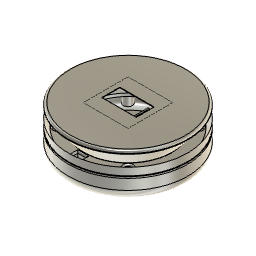
IR Hub v26 (Autodesk Fusion 360 design; units mm, degrees)
Autodesk Fusion 360 part; units mm, degrees
note: some values were not read from the file. Set by a fixed rule: which sketch regions a step uses.
sketch "Sketch1" plane through (0, 0, 0) normal (0, 1, 0) x (1, 0, 0)
  line L0 (0, 0) -> (0, -2) construction
  line L1 (0, -2) -> (33, -2)
  line L2 (38, -7) -> (38, -14)
  line L3 (0, -2) -> (0, 0)
  line L4 (38, -14) -> (40, -14)
  arc A0 (38, -7) -> (33, -2) centre (33, -7) ccw
  line L5 (0, 0) -> (33, 0)
  arc A1 (40, -7) -> (33, 0) centre (33, -7) ccw
  line L6 (40, -7) -> (40, -14)
  line L7 (0, 0) -> (80, 0)
  line L8 (80, 0) -> (80, -14)
  line L9 (40, -14) -> (80, -14)
  point P0 (38, -2)
  dimension "d5" = 2
  dimension "d6" = 38
  dimension "d7" = 12
  dimension "d9" = 5
  dimension "d40" = 80
  dimension "d41" = 14
  constraint coincident L0.start L3.end
  constraint vertical L0
  constraint perpendicular L0 L1
  constraint perpendicular L1 L2
  constraint perpendicular L3 L5
  constraint perpendicular L4 L6
  constraint coincident P0 L1
  constraint coincident P0 L2
  constraint tangent L1 A0
  constraint tangent L2 A0
  constraint perpendicular L3 L7
  constraint perpendicular L5 L8
  measures "d5" distance of L0.start L0.end
  measures "d6" distance of L0.end P0
  measures "d7" distance of P0 L2.end
  measures "d9" radius of A0
  measures "d40" distance of L0.start L7.end
  measures "d41" distance of L7.end L8.end
revolve "Revolve1" add sketch "Sketch1" angle 360 about axis through (0, 0, 1.75) along (0, 0, 1) contours L1 L2 L3 L4 A0 L5 A1 L6 L7 makes body 1
sketch "Sketch2" plane through (0, 0, 2) normal (0, 0, 1) x (-1, 0, 0)
  circle A0 centre (0, 0) radius 33
  line L0 (-16, -29.5) -> (16, -29.5)
  line L1 (16, -29.5) -> (16, 29.5)
  line L2 (16, 29.5) -> (-16, 29.5)
  line L3 (-16, 29.5) -> (-16, -29.5)
  line L4 (-16, -29.5) -> (16, 29.5) construction
  line L5 (16, -29.5) -> (-16, 29.5) construction
  line L6 (-17, 30.5) -> (-17, -30.5)
  line L7 (-17, -30.5) -> (17, -30.5)
  line L8 (17, -30.5) -> (17, 30.5)
  line L9 (17, 30.5) -> (-17, 30.5)
  dimension "d16" = 32
  dimension "d17" = 59
  dimension "d20" = 1
  constraint horizontal L0
  constraint perpendicular L0 L1
  constraint parallel L0 L2
  constraint parallel L1 L3
  constraint coincident L4 A0.centre
  constraint coincident L5 A0.centre
  constraint coincident A0.centre origin
  measures "d16" distance of L1.end L2.end
  measures "d17" distance of L0.end L1.end
extrude "Extrude1" add sketch "Sketch2" along normal blind 1 contours A0 L1 L8 | A0 L1 L2 L8 L9 | A0 L0 L1 L7 L8 | A0 L2 L9 | A0 L0 L7 | A0 L2 L3 L6 L9 | A0 L0 L3 L6 L7 | A0 L3 L6 bodies 1
sketch "Sketch3" plane through (0, 30.5, 0) normal (0, 1, 0) x (-1, 0, 0)
  line L0 (17, 3) -> (-17, 3)
  line L1 (0, 2) -> (0, 5.5) construction
  line L2 (4.5, 7.5) -> (-4.5, 7.5)
  line L3 (-4.5, 7.5) -> (-4.5, 3.5)
  line L4 (-4.5, 3.5) -> (4.5, 3.5)
  line L5 (4.5, 3.5) -> (4.5, 7.5)
  line L6 (4.5, 7.5) -> (-4.5, 3.5) construction
  line L7 (-4.5, 7.5) -> (4.5, 3.5) construction
  line L8 (7.5, 9.5) -> (-7.5, 9.5)
  line L9 (-7.5, 9.5) -> (-7.5, 1.5)
  line L10 (-7.5, 1.5) -> (7.5, 1.5)
  line L11 (7.5, 1.5) -> (7.5, 9.5)
  line L12 (7.5, 9.5) -> (-7.5, 1.5) construction
  line L13 (-7.5, 9.5) -> (7.5, 1.5) construction
  line L14 (8.5, 1.5) -> (8.5, 10.5)
  line L15 (8.5, 10.5) -> (-8.5, 10.5)
  line L16 (-8.5, 10.5) -> (-8.5, 1.5)
  line L17 (-8.5, 1.5) -> (-7.5, 1.5)
  line L18 (8.5, 1.5) -> (7.5, 1.5)
  spline S0 degree 3 poles (17, 2.3824) (16.4779, 2.2768) (15.935, 2.1958) (14.4367, 2.0345) (13.4748, 2) (12.5996, 2) knots -1.596795 -1.596795 -1.596795 -1.596795 -1.446279 -1.446279 -1.183716 -1.183716 -1.183716 -1.183716
  line L19 (17, 2.3824) -> (17, 3)
  line L20 (-17, 3) -> (-17, 2.3824)
  spline S1 degree 3 poles (-12.5996, 2) (-13.4748, 2) (-14.4367, 2.0345) (-15.935, 2.1958) (-16.4779, 2.2768) (-17, 2.3824) knots 1.183716 1.183716 1.183716 1.183716 1.446279 1.446279 1.596795 1.596795 1.596795 1.596795
  line L21 (-12.5996, 2) -> (12.5996, 2)
  point P0 (0, 5.5)
  point P1 (0, 5.5)
  dimension "d23" = 3.5
  dimension "d24" = 9
  dimension "d25" = 4
  dimension "d29" = 15
  dimension "d30" = 8
  dimension "d31" = 1
  constraint perpendicular L0 L1
  constraint horizontal L2
  constraint perpendicular L2 L3
  constraint parallel L2 L4
  constraint parallel L3 L5
  constraint coincident L6 P1
  constraint coincident L7 P1
  constraint coincident P1 P0
  constraint horizontal L8
  constraint perpendicular L8 L9
  constraint parallel L8 L10
  constraint parallel L9 L11
  constraint coincident L12 P1
  constraint coincident L13 P1
  constraint perpendicular L9 L17
  constraint perpendicular L11 L18
  measures "d23" distance of L1.start P1
  measures "d24" distance of L3.end L4.end
  measures "d25" distance of L2.end L3.end
  measures "d29" distance of L9.end L10.end
  measures "d30" distance of L8.end L9.end
extrude "Extrude2" cut sketch "Sketch3" along normal blind 80 contours L0 L9 L11 L21 | L0 L8 L9 L11 | L9 L10 L11 L21 | L2 L3 L4 L5 bodies 1
extrude "Extrude3" add sketch "Sketch3" along normal blind 16.314 contours L0 L11 L14 L21 | L0 L8 L9 L11 L14 L15 L16 | L0 L9 L16 L21 bodies 1
extrude "Extrude4" add sketch "Sketch3" along normal blind 1 separate body contours L0 L8 L9 L11 makes body 2
extrude "Extrude5" add 1 faces at (-2.5, 30.5, 2) along direction (0, 1, 0) blind 1 on bodies 1 bodies 1 2
revolve "Revolve2" cut sketch "Sketch1" angle 360 about axis through (0, 0, 1.75) along (0, 0, 1) contours A1 L6 L7 L8 L9 bodies 1
sketch "Sketch4" plane through (0, 0, 0) normal (0, 0, 1) x (1, 0, 0)
  circle A0 centre (0, 0) radius 40
  circle A1 centre (0, 0) radius 37.6
  circle A2 centre (0, 0) radius 36.6
  line L0 (23.5, 23.5) -> (-23.5, 23.5) construction
  line L1 (-23.5, 23.5) -> (-23.5, -23.5) construction
  line L2 (-23.5, -23.5) -> (23.5, -23.5) construction
  line L3 (23.5, -23.5) -> (23.5, 23.5) construction
  line L4 (23.5, 23.5) -> (-23.5, -23.5) construction
  line L5 (-23.5, 23.5) -> (23.5, -23.5) construction
  circle A3 centre (23.5, 23.5) radius 2.5
  circle A4 centre (23.5, -23.5) radius 2.5
  circle A5 centre (-23.5, -23.5) radius 2.5
  circle A6 centre (-23.5, 23.5) radius 2.5
  circle A7 centre (-23.5, 23.5) radius 3
  circle A8 centre (23.5, 23.5) radius 3
  circle A9 centre (23.5, -23.5) radius 3
  circle A10 centre (-23.5, -23.5) radius 3
  line L6 (0, 0) -> (0, -33.234) construction
  line L7 (2.75, -30.984) -> (-2.75, -30.984)
  line L8 (-2.75, -30.984) -> (-2.75, -35.484)
  line L9 (-2.75, -35.484) -> (2.75, -35.484)
  line L10 (2.75, -35.484) -> (2.75, -30.984)
  line L11 (2.75, -30.984) -> (-2.75, -35.484) construction
  line L12 (-2.75, -30.984) -> (2.75, -35.484) construction
  line L13 (-3.25, -30.484) -> (-3.25, -35.984)
  line L14 (-3.25, -35.984) -> (3.25, -35.984)
  line L15 (3.25, -35.984) -> (3.25, -30.484)
  line L16 (3.25, -30.484) -> (-3.25, -30.484)
  circle A11 centre (0, 0) radius 29.5
  point P0 (0, -33.234)
  dimension "d43" = 80
  dimension "d50" = 47
  dimension "d51" = 47
  dimension "d53" = 5
  dimension "d54" = 5
  dimension "d55" = 5
  dimension "d56" = 5
  dimension "d58" = 0.5
  dimension "d59" = 0.5
  dimension "d60" = 0.5
  dimension "d61" = 0.5
  dimension "d65" = 33.234
  dimension "d66" = 5.5
  dimension "d67" = 4.5
  dimension "d68" = 0.5
  dimension "d70" = 59
  constraint coincident A0.centre A1.centre
  constraint horizontal L0
  constraint perpendicular L0 L1
  constraint parallel L0 L2
  constraint parallel L1 L3
  constraint coincident L4 A0.centre
  constraint coincident L5 A0.centre
  constraint coincident L0.start L3.end
  constraint coincident L2.end L3.start
  constraint coincident L1.end L2.start
  constraint coincident L0.end L1.start
  constraint vertical L6
  constraint horizontal L7
  constraint perpendicular L7 L8
  constraint parallel L7 L9
  constraint parallel L8 L10
  constraint coincident L11 P0
  constraint coincident L12 P0
  constraint coincident P0 L6.end
  measures "d43" diameter of A0
  measures "d50" distance of L1.end L2.end
  measures "d51" distance of L0.end L1.end
  measures "d53" diameter of A3
  measures "d54" diameter of A4
  measures "d55" diameter of A5
  measures "d56" diameter of A6
  measures "d65" distance of A0.centre P0
  measures "d66" distance of L8.end L9.end
  measures "d67" distance of L7.end L8.end
  measures "d70" diameter of A11
extrude "Extrude6" add sketch "Sketch4" along normal blind 1.5 separate body contours A0 | A1 | A2 makes body 3
extrude "Extrude7" add sketch "Sketch4" along normal blind 2.5 contours A1 bodies 3
extrude "Extrude8" add sketch "Sketch4" along normal blind 9.5 contours A7 | A8 | A9 | A10 bodies 3
extrude "Extrude9" add sketch "Sketch4" along normal blind 9.5 contours L13 L14 L15 L16 bodies 3
fillet "Fillet1" radius 1 8 edges at (21.1692, 24.404, 0) (21.1692, -22.596, 0) (0, -30.984, 0) (-2.75, -33.234, 0) (0, -35.484, 0) (2.75, -33.234, 0) (-25.8308, -22.596, 0) (-25.8308, 24.404, 0) on bodies 3
fillet "Fillet2" radius 0.5 1 edges at (-37.2931, -14.4646, 0) on bodies 3
sketch "Sketch5" plane through (0, 0, 0) normal (0, 1, 0) x (1, 0, 0)
  line L0 (0, 0) -> (29.5, 0) construction
  line L1 (29.5, 0) -> (40, -12.5134)
  line L2 (29.5, 0) -> (37.5, 0) construction
  line L3 (29.5, 0) -> (29, 0)
  line L4 (29, 0) -> (29, 2)
  line L5 (40, -12.5134) -> (40, 0) construction
  line L6 (40, -12.5134) -> (38.5, -12.5134)
  line L7 (38.5, -12.5134) -> (28, 0)
  line L8 (38.5, -12.5134) -> (60.6777, -12.5134) construction
  line L9 (28, 0) -> (28, 2)
  line L10 (28, 2) -> (29, 2)
  dimension "d88" = 29.5
  dimension "d89" = 50
  dimension "d90" = 16.3351
  dimension "d93" = 0.5
  dimension "d95" = 2
  dimension "d97" = 1.5
  dimension "d98" = 130
  dimension "d99" = 2
  constraint coincident L0.start origin
  constraint horizontal L0
  constraint horizontal L2
  constraint parallel L0 L3
  constraint perpendicular L0 L4
  constraint horizontal L6
  constraint perpendicular L5 L6
  constraint horizontal L8
  constraint coincident L0 L7.end
  constraint perpendicular L0 L9
  measures "d88" distance of L0.start L0.end
  measures "d89" angle of L1 L2
  measures "d90" distance of L0.end L1.end
  measures "d93" distance of L0.end L3.end
  measures "d95" distance of L3.end L4.end
  measures "d97" distance of L1.end L6.end
  measures "d98" angle of L7 L8
  measures "d99" distance of L7.end L9.end
revolve "Revolve3" add sketch "Sketch5" angle 360 about axis through (0, 0, 1.75) along (0, 0, 1) separate body makes body 4
move_body "Move1" bodies 4 to x (1, 0, 0) y (0, 1, 0) z (0, 0, 1) at (0, 0, 2)
move_body "Move2" bodies 4 to x (1, 0, 0) y (0, 1, 0) z (0, 0, 1) at (0, 0, 50)
move_body "Move3" bodies 3 to x (-1, 0, 0) y (0, 1, 0) z (0, 0, -1) at (0, 0, 34)
move_body "Move4" bodies 3 to x (1, 0, 0) y (0, 1, 0) z (0, 0, 1) at (0, 0, -10.5)
move_body "Move5" bodies 4 to x (1, 0, 0) y (0, 1, 0) z (0, 0, 1) at (0, 0, -28.5)
move_body "Move6" bodies 4 3 to x (1, 0, 0) y (0, 1, 0) z (0, 0, 1) at (0, 0, -5)
sketch "Sketch6" plane through (0, 0, 0) normal (0, 1, 0) x (1, 0, 0)
  line L0 (0, 0) -> (38.5, 0)
  line L1 (40, -1.5) -> (40, -2)
  line L2 (40, -2) -> (0, -2)
  line L3 (0, -2) -> (0, 0)
  line L4 (40, -2) -> (38.3, -2) construction
  line L5 (38.3, -2) -> (37.0144, -3.5321)
  line L6 (38.3, -2) -> (45, -2) construction
  line L7 (37.0144, -3.5321) -> (37.0144, -2)
  arc A0 (40, -1.5) -> (38.5, 0) centre (38.5, -1.5) ccw
  point P0 (40, 0)
  dimension "d101" = 40
  dimension "d102" = 2
  dimension "d105" = 1.7
  dimension "d106" = 130
  dimension "d107" = 2
  dimension "d109" = 1.5
  constraint horizontal L0
  constraint vertical L1
  constraint horizontal L2
  constraint vertical L3
  constraint coincident L0.start L3.end
  constraint perpendicular L1 L4
  constraint horizontal L6
  constraint coincident L2 L7.end
  constraint perpendicular L2 L7
  constraint coincident P0 L0
  constraint coincident P0 L1
  constraint tangent L0 A0
  constraint tangent L1 A0
  measures "d101" distance of L0.start P0
  measures "d102" distance of L0.start L2.end
  measures "d105" distance of L1.end L4.end
  measures "d106" angle of L5 L6
  measures "d107" distance of L4.end L5.end
  measures "d109" radius of A0
revolve "Revolve4" add sketch "Sketch6" angle 360 about axis through (0, 0, 1.75) along (0, 0, 1) separate body makes body 5
sketch "Sketch7" plane through (0, 0, 2) normal (0, 0, 1) x (-1, 0, 0)
  circle A0 centre (0, 0) radius 37.0144
  line L0 (-15, -15) -> (15, -15)
  line L1 (15, -15) -> (15, 15)
  line L2 (15, 15) -> (-15, 15)
  line L3 (-15, 15) -> (-15, -15)
  line L4 (-15, -15) -> (15, 15) construction
  line L5 (15, -15) -> (-15, 15) construction
  line L6 (-11.5, -6) -> (11.5, -6)
  line L7 (11.5, -6) -> (11.5, 6)
  line L8 (11.5, 6) -> (-11.5, 6)
  line L9 (-11.5, 6) -> (-11.5, -6)
  line L10 (-11.5, -6) -> (11.5, 6) construction
  line L11 (11.5, -6) -> (-11.5, 6) construction
  dimension "d114" = 30
  dimension "d115" = 30
  dimension "d116" = 23
  dimension "d117" = 12
  constraint horizontal L0
  constraint perpendicular L0 L1
  constraint parallel L0 L2
  constraint parallel L1 L3
  constraint coincident L4 A0.centre
  constraint coincident L5 A0.centre
  constraint coincident A0.centre origin
  constraint horizontal L6
  constraint perpendicular L6 L7
  constraint parallel L6 L8
  constraint parallel L7 L9
  constraint coincident L10 A0.centre
  constraint coincident L11 A0.centre
  measures "d114" distance of L1.end L2.end
  measures "d115" distance of L0.end L1.end
  measures "d116" distance of L7.end L8.end
  measures "d117" distance of L6.end L7.end
extrude "Extrude10" cut sketch "Sketch7" against normal blind 2 contours L6 L7 L8 L9 bodies 5
extrude "Extrude11" cut sketch "Sketch7" against normal blind 1.6 contours L0 L1 L2 L3 bodies 5
move_body "Move7" bodies 5 to x (-1, 0, 0) y (0, 1, 0) z (0, 0, -1) at (0, 0, 33)
move_body "Move8" bodies 5 4 3 to x (1, 0, 0) y (0, 1, 0) z (0, 0, 1) at (0, 0, -3)
sketch "Sketch8" plane through (0, 0, 0) normal (0, 1, 0) x (1, 0, 0)
  line L0 (0, 0) -> (40, 0) construction
  line L1 (40, 0) -> (40, -5)
  line L2 (40, 0) -> (37, 0)
  line L3 (37, 0) -> (40, -5)
  dimension "d125" = 40
  dimension "d126" = 5
  dimension "d127" = 3
  constraint coincident L0.start origin
  constraint horizontal L0
  constraint perpendicular L0 L1
  constraint perpendicular L1 L2
  measures "d125" distance of L0.start L0.end
  measures "d126" distance of L0.end L1.end
  measures "d127" distance of L0.end L2.end
revolve "Revolve5" add sketch "Sketch8" angle 360 about axis through (0, 0, 1.75) along (0, 0, 1) separate body makes body 6
move_body "Move9" bodies 6 to x (1, 0, 0) y (0, 1, 0) z (0, 0, 1) at (0, 0, 15)
move_body "Move10" bodies 6 to x (1, 0, 0) y (0, 1, 0) z (0, 0, 1) at (0, 0, 0.5)
equation "base_thickness = 2 mm"
equation "base_dia = 80 mm"
equation "base_curve = 5 mm"
equation "base_height = 12 mm"
equation "d5 = base_thickness"
equation "d6 = base_dia / 2 - base_thickness"
equation "d7 = base_height"
equation "d8 = -base_thickness"
equation "d9 = base_curve"
equation "mcu_len = 59 mm"
equation "mcu_width = 32 mm"
equation "mcu_port_offset_y = 1.5 mm"
equation "mcu_port_len = 9 mm"
equation "mcu_port_width = 4 mm"
equation "d16 = mcu_width"
equation "d17 = mcu_len"
equation "mcu_support_thickness = 1 mm"
equation "mcu_support_height = 1 mm"
equation "d20 = mcu_support_thickness"
equation "d21 = mcu_support_height"
equation "d23 = mcu_port_offset_y + mcu_port_width / 2"
equation "d24 = mcu_port_len"
equation "d25 = mcu_port_width"
equation "base_port_hole_len = 15 mm"
equation "base_port_hole_width = 8 mm"
equation "base_port_thickness = 1 mm"
equation "d29 = base_port_hole_len"
equation "d30 = base_port_hole_width"
equation "d31 = base_port_thickness"
equation "d32 = base_dia"
equation "d36 = base_port_thickness"
equation "d38 = base_port_thickness"
equation "d40 = base_dia"
equation "d41 = base_height + base_thickness"
equation "d43 = base_dia"
equation "join_thickness = 1 mm"
equation "join_offset = 0.4 mm"
equation "d46 = -join_offset - base_thickness"
equation "d47 = -join_offset - join_thickness - base_thickness"
equation "ir_array_len = 47 mm"
equation "ir_dia = 5 mm"
equation "d50 = ir_array_len"
equation "d51 = ir_array_len"
equation "ir_len = 8 mm"
equation "d53 = ir_dia"
equation "d54 = ir_dia"
equation "d55 = ir_dia"
equation "d56 = ir_dia"
equation "ir_channel_thickness = 0.5 mm"
equation "d58 = ir_channel_thickness"
equation "d59 = ir_channel_thickness"
equation "d60 = ir_channel_thickness"
equation "d61 = ir_channel_thickness"
equation "ir_rx_len = 5.5 mm"
equation "ir_rx_width = 4.5 mm"
equation "ir_rx_height = 8 mm"
equation "d65 = ir_array_len / sqrt(2)"
equation "d66 = ir_rx_len"
equation "d67 = ir_rx_width"
equation "d68 = ir_channel_thickness"
equation "base_center_hole_dia = 59 mm"
equation "d70 = base_center_hole_dia"
equation "base_cover_thickness = 1.5 mm"
equation "d72 = base_cover_thickness"
equation "d74 = base_cover_thickness + join_thickness"
equation "d76 = ir_len + base_cover_thickness"
equation "d78 = base_cover_thickness + ir_rx_height"
equation "ir_chamfer = 1 mm"
equation "d82 = ir_chamfer"
equation "base_top_chamfer = 0.5 mm"
equation "d85 = base_top_chamfer"
equation "ctr_angle = 50 deg"
equation "ctr_height = 10 mm"
equation "d88 = base_center_hole_dia / 2"
equation "d89 = ctr_angle"
equation "d90 = ( base_dia / 2 - base_center_hole_dia / 2 ) / cos(ctr_angle)"
equation "ctr_thickness = 1.5 mm"
equation "ctr_hole_offset = 0.5 mm"
equation "d93 = ctr_hole_offset"
equation "ctr_join_thickness = 2 mm"
equation "d95 = ctr_join_thickness"
equation "d97 = ctr_thickness"
equation "d98 = 180 deg - ctr_angle"
equation "d99 = ctr_join_thickness"
equation "d101 = base_dia / 2"
equation "d102 = base_thickness"
equation "top_join_thickness = 2 mm"
equation "top_join_offset = ctr_thickness + 0.2 mm"
equation "d105 = top_join_offset"
equation "d106 = 180 deg - ctr_angle"
equation "d107 = top_join_thickness"
equation "top_chamfer = 1.5 mm"
equation "d109 = top_chamfer"
equation "display_out_len = 30 mm"
equation "display_len = 23 mm"
equation "display_width = 12 mm"
equation "d114 = display_out_len"
equation "d115 = display_out_len"
equation "d116 = display_len"
equation "d117 = display_width"
equation "d118 = -base_thickness"
equation "display_cover_thickness = 0.4 mm"
equation "d121 = display_cover_thickness - base_thickness"
equation "guide_len = 3 mm"
equation "guide_height = 5 mm"
equation "d125 = base_dia / 2"
equation "d126 = guide_height"
equation "d127 = guide_len"
named bodies: "Base", "Led Holder", "Inner Guide", "Top", "Outer Guide"
